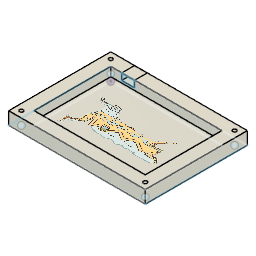
macropad cad files (Autodesk Fusion 360 design; units mm, degrees)
part number: 2026-06-19-12-53-12-987
Autodesk Fusion 360 part; units mm, degrees
sketch "Sketch1" plane through (0, 0, 0) normal (0, 1, 0) x (1, 0, 0)
  line L0 (0, 0) -> (87, 0)
  line L1 (87, 0) -> (87, -60)
  line L2 (87, -60) -> (0, -60)
  line L3 (0, -60) -> (0, 0)
  line L4 (-10, 10) -> (97, 10)
  line L5 (97, 10) -> (97, -70)
  line L6 (97, -70) -> (-10, -70)
  line L7 (-10, -70) -> (-10, 10)
  circle A0 centre (-5, 5) radius 1.45
  circle A1 centre (-5, -65) radius 1.45
  circle A2 centre (92, -65) radius 1.45
  circle A3 centre (92, 5) radius 1.45
  dimension "d1" = 87
  dimension "d2" = 60
  dimension "d3" = 107
  dimension "d4" = 80
  dimension "d5" = 10
  dimension "d6" = 2.9
  dimension "d7" = 5
  dimension "d8" = 2.9
  dimension "d9" = 5
  dimension "d10" = 5
  dimension "d11" = 2.9
  dimension "d12" = 5
  dimension "d13" = 5
  dimension "d14" = 2.9
  dimension "d15" = 5
  dimension "d16" = 5
  constraint horizontal L0
  constraint vertical L1
  constraint horizontal L2
  constraint vertical L3
  constraint coincident L0.start L3.end
  constraint horizontal L4
  constraint vertical L5
  constraint horizontal L6
  constraint vertical L7
  measures "d1" distance of L0.start L0.end
  measures "d2" distance of L0.start L2.end
  measures "d3" distance of L4.start L4.end
  measures "d4" distance of L4.start L6.end
  measures "d5" distance of L2 L6
  measures "d6" diameter of A0
  measures "d7" distance of L7 A0.centre
  measures "d8" diameter of A1
  measures "d9" distance of L7 A1.centre
  measures "d10" distance of L2 A1.centre
  measures "d11" diameter of A2
  measures "d12" distance of L2 A2.centre
  measures "d13" distance of L5 A2.centre
  measures "d14" diameter of A3
  measures "d15" distance of L4 A3.centre
  measures "d16" distance of L5 A3.centre
extrude "Extrude1" add sketch "Sketch1" along normal blind 3 contours L0 L1 L2 L3 | L4 L5 L6 L7
extrude "Extrude2" cut sketch "Sketch1" along normal blind 10
extrude "Extrude3" add sketch "Sketch1" along normal blind 10
sketch "Sketch3" plane through (0, 0, 0) normal (0, 0, 1) x (1, 0, 0)
  line L0 (8.5266, 9.753) -> (18.5266, 9.753)
  line L1 (18.5266, 9.753) -> (18.5266, 4.753)
  line L2 (18.5266, 4.753) -> (8.5266, 4.753)
  line L3 (8.5266, 4.753) -> (8.5266, 9.753)
  dimension "d23" = 10
  dimension "d24" = 5
  constraint horizontal L0
  constraint vertical L1
  constraint horizontal L2
  constraint vertical L3
  measures "d23" distance of L0.start L0.end
  measures "d24" distance of L0.start L2.end
extrude "Extrude4" cut sketch "Sketch3" against normal blind 10
